Autodesk Fusion 360 part; units mm, degrees
note: some values were not read from the file. Set by a fixed rule: which face or edge a step refers to.
(part 2 of 4)
sketch "Sketch39" plane through (-432.6941, 0, 0) normal (-1, 0, 0) x (0, -1, 0)
  circle A0 centre (25, -180) radius 4
  circle A1 centre (50, 175) radius 4
  circle A2 centre (25, 170) radius 4
  circle A3 centre (50, -175) radius 4
  circle A4 centre (75, 180) radius 4
  circle A5 centre (75, -170) radius 4
  arc A6 (0, 125.6014) -> (0, 130.6014) centre (0, 128.1014) ccw
  line L0 (0, 125.6014) -> (-10, 125.6014)
  line L1 (-10, 125.6014) -> (-10, 18.1014)
  line L2 (-10, 18.1014) -> (0, 18.1014)
  arc A7 (0, 13.1014) -> (0, 18.1014) centre (0, 15.6014) ccw
  line L3 (0, 13.1014) -> (0, -6.8986)
  arc A8 (0, -11.8986) -> (0, -6.8986) centre (0, -9.3986) ccw
  line L4 (0, -11.8986) -> (-10, -11.8986)
  line L5 (-10, -11.8986) -> (-10, -119.3986)
  line L6 (-10, -119.3986) -> (0, -119.3986)
  arc A9 (0, -124.3986) -> (0, -119.3986) centre (0, -121.8986) ccw
  line L7 (0, -124.3986) -> (0, -144.3986)
  arc A10 (0, -149.3986) -> (0, -144.3986) centre (0, -146.8986) ccw
  line L8 (0, -149.3986) -> (-10, -149.3986)
  line L9 (-10, -149.3986) -> (-10, -256.3488)
  line L10 (-10, -256.3488) -> (30, -256.3488)
  line L11 (30, -256.3488) -> (30, -246.3488)
  arc A11 (35, -246.3488) -> (30, -246.3488) centre (32.5, -246.3488) ccw
  line L12 (35, -246.3488) -> (55, -246.3488)
  arc A12 (60, -246.3488) -> (55, -246.3488) centre (57.5, -246.3488) ccw
  line L13 (60, -246.3488) -> (60, -256.3488)
  line L14 (60, -256.3488) -> (100, -256.3488)
  line L15 (100, -256.3488) -> (100, 273.6512)
  line L16 (100, 273.6512) -> (60, 273.6512)
  line L17 (60, 273.6512) -> (60, 263.6512)
  arc A13 (55, 263.6512) -> (60, 263.6512) centre (57.5, 263.6512) ccw
  line L18 (55, 263.6512) -> (35, 263.6512)
  arc A14 (30, 263.6512) -> (35, 263.6512) centre (32.5, 263.6512) ccw
  line L19 (30, 263.6512) -> (30, 273.6512)
  line L20 (30, 273.6512) -> (-10, 273.6512)
  line L21 (-10, 273.6512) -> (-10, 155.6014)
  line L22 (-10, 155.6014) -> (0, 155.6014)
  arc A15 (0, 150.6014) -> (0, 155.6014) centre (0, 153.1014) ccw
  line L23 (0, 150.6014) -> (0, 140.6014)
  arc A16 (0, 135.6014) -> (0, 140.6014) centre (0, 138.1014) ccw
  line L24 (0, 135.6014) -> (0, 130.6014)
  line L25 (0, 140.6014) -> (2.5, 140.6014)
  line L26 (2.5, 140.6014) -> (2.5, 134.5426)
  line L27 (2.5, 134.5426) -> (0, 134.5426)
  line L28 (0, 134.5426) -> (0, 140.6014)
  constraint horizontal L25
  constraint vertical L26
  constraint horizontal L27
  constraint vertical L28
  constraint coincident L23.end A16.end
extrude "Extrude20" add sketch "Sketch39" against normal blind 10 contours A16 L28 bodies 3
sketch "Sketch40" plane through (-142.6941, 0, 0) normal (-1, 0, 0) x (0, -1, 0)
  line L0 (0, 135.6014) -> (0, 130.6014)
  arc A0 (0, 125.6014) -> (0, 130.6014) centre (0, 128.1014) ccw
  line L1 (0, 125.6014) -> (-10, 125.6014)
  line L2 (-10, 125.6014) -> (-10, 18.1014)
  line L3 (-10, 18.1014) -> (0, 18.1014)
  arc A1 (0, 13.1014) -> (0, 18.1014) centre (0, 15.6014) ccw
  line L4 (0, 13.1014) -> (0, -6.8986)
  arc A2 (0, -11.8986) -> (0, -6.8986) centre (0, -9.3986) ccw
  line L5 (0, -11.8986) -> (-10, -11.8986)
  line L6 (-10, -11.8986) -> (-10, -119.3986)
  line L7 (-10, -119.3986) -> (0, -119.3986)
  arc A3 (0, -124.3986) -> (0, -119.3986) centre (0, -121.8986) ccw
  line L8 (0, -124.3986) -> (0, -144.3986)
  arc A4 (0, -149.3986) -> (0, -144.3986) centre (0, -146.8986) ccw
  line L9 (0, -149.3986) -> (-10, -149.3986)
  line L10 (-10, -149.3986) -> (-10, -256.3488)
  line L11 (-10, -256.3488) -> (30, -256.3488)
  line L12 (30, -256.3488) -> (30, -246.3488)
  arc A5 (35, -246.3488) -> (30, -246.3488) centre (32.5, -246.3488) ccw
  line L13 (35, -246.3488) -> (55, -246.3488)
  arc A6 (60, -246.3488) -> (55, -246.3488) centre (57.5, -246.3488) ccw
  line L14 (60, -246.3488) -> (60, -256.3488)
  line L15 (60, -256.3488) -> (100, -256.3488)
  line L16 (100, -256.3488) -> (100, 273.6512)
  line L17 (100, 273.6512) -> (60, 273.6512)
  line L18 (60, 273.6512) -> (60, 263.6512)
  arc A7 (55, 263.6512) -> (60, 263.6512) centre (57.5, 263.6512) ccw
  line L19 (55, 263.6512) -> (35, 263.6512)
  arc A8 (30, 263.6512) -> (35, 263.6512) centre (32.5, 263.6512) ccw
  line L20 (30, 263.6512) -> (30, 273.6512)
  line L21 (30, 273.6512) -> (-10, 273.6512)
  line L22 (-10, 273.6512) -> (-10, 155.6014)
  line L23 (-10, 155.6014) -> (0, 155.6014)
  arc A9 (0, 150.6014) -> (0, 155.6014) centre (0, 153.1014) ccw
  line L24 (0, 150.6014) -> (0, 140.6014)
  arc A10 (0, 135.6014) -> (0, 140.6014) centre (0, 138.1014) ccw
  circle A11 centre (75, -170) radius 4
  circle A12 centre (75, 180) radius 4
  circle A13 centre (50, -175) radius 4
  circle A14 centre (25, 170) radius 4
  circle A15 centre (50, 175) radius 4
  circle A16 centre (25, -180) radius 4
  line L25 (0, 140.6014) -> (7, 140.6014)
  line L26 (7, 140.6014) -> (7, 132.6014)
  line L27 (7, 132.6014) -> (0, 132.6014)
  line L28 (0, 132.6014) -> (0, 140.6014)
  constraint horizontal L25
  constraint vertical L26
  constraint horizontal L27
  constraint vertical L28
  constraint coincident L24.end A10.end
extrude "Extrude21" add sketch "Sketch40" against normal blind 10 contours A10 L28 bodies 2
sketch "Sketch41" plane through (0, 0, 0) normal (0, -1, 0) x (1, 0, 0)
  line L0 (-332.6941, 163.1014) -> (-342.6941, 163.1014)
  line L1 (-342.6941, 163.1014) -> (-342.6941, 213.1014)
  line L2 (-342.6941, 213.1014) -> (-332.6941, 213.1014)
  line L3 (-332.6941, 213.1014) -> (-332.6941, 163.1014)
  point P0 (-332.6941, 163.1014)
  dimension "d245" = 10
  dimension "d246" = 50
  constraint horizontal L0
  constraint vertical L1
  constraint horizontal L2
  constraint vertical L3
  constraint coincident P0 L0.start
  measures "d245" distance of P0 L0.end
  measures "d246" distance of P0 L2.end
extrude "Extrude22" add sketch "Sketch41" along normal blind 70 separate body makes body 5
sketch "Sketch42" plane through (-332.6941, 0, 0) normal (1, 0, 0) x (0, 1, 0)
  line L0 (0, 163.1014) -> (0, 213.1014)
  line L1 (0, 213.1014) -> (-70, 213.1014)
  line L2 (-70, 213.1014) -> (-70, 163.1014)
  line L3 (-70, 163.1014) -> (0, 163.1014)
  line L4 (0, 198.1014) -> (10, 198.1014)
  line L5 (10, 198.1014) -> (10, 178.1014)
  line L6 (10, 178.1014) -> (0, 178.1014)
  line L7 (0, 178.1014) -> (0, 198.1014)
  line L8 (0, 193.1014) -> (0, 183.1014)
  line L9 (-70, 223.1014) -> (-65, 223.1014)
  line L10 (-65, 223.1014) -> (-65, 213.1014)
  line L11 (-65, 213.1014) -> (-70, 213.1014)
  line L12 (-70, 213.1014) -> (-70, 223.1014)
  dimension "d249" = 10
  dimension "d250" = 20
  dimension "d251" = 5
  dimension "d252" = 10
  constraint horizontal L4
  constraint vertical L5
  constraint horizontal L6
  constraint vertical L7
  constraint midpoint L7 L8
  constraint horizontal L9
  constraint vertical L10
  constraint horizontal L11
  constraint vertical L12
  constraint coincident L1.end L2.start
  measures "d249" distance of L4.start L4.end
  measures "d250" distance of L4.start L6.end
  measures "d251" distance of L9.start L9.end
  measures "d252" distance of L9.start L1.end
extrude "Extrude23" add sketch "Sketch42" against normal blind 10 contours L0 L4 L5 L6 L7 L8 | L1 L9 L10 L11 L12 bodies 5
sketch "Sketch43" plane through (-332.6941, 0, 0) normal (1, 0, 0) x (0, 1, 0)
  line L0 (0, 198.1014) -> (0, 213.1014)
  line L1 (0, 213.1014) -> (-65, 213.1014)
  line L2 (-65, 213.1014) -> (-65, 223.1014)
  line L3 (-65, 223.1014) -> (-70, 223.1014)
  line L4 (-70, 223.1014) -> (-70, 163.1014)
  line L5 (-70, 163.1014) -> (0, 163.1014)
  line L6 (0, 163.1014) -> (0, 178.1014)
  line L7 (0, 178.1014) -> (10, 178.1014)
  line L8 (10, 178.1014) -> (10, 198.1014)
  line L9 (10, 198.1014) -> (0, 198.1014)
  circle A0 centre (0, 200.6014) radius 2.5
  circle A1 centre (0, 175.6014) radius 2.5
  circle A2 centre (-62.5, 213.1014) radius 2.5
  line L10 (-5.4259, 163.1014) -> (-70, 190)
  line L11 (-70, 163.1014) -> (-70, 190)
  line L12 (-70, 163.1014) -> (-5.4259, 163.1014)
  dimension "d255" = 5
  dimension "d256" = 5
  dimension "d257" = 5
  constraint coincident L0.start A0
  constraint coincident L6.end A1
  constraint coincident L1.end A2
  constraint coincident L5 L10.start
  constraint coincident L4 L10.end
  constraint coincident L4.end L5.start
  measures "d255" diameter of A0
  measures "d256" diameter of A1
  measures "d257" diameter of A2
extrude "Extrude24" cut sketch "Sketch43" against normal blind 10 contours L0 A0 | L1 A2 | L6 A1 | L4 L5 L10 L11 L12 picked at (-0.8152, 201.2122) picked at (-62.5623, 212.2704) picked at (-0.8999, 175.0818) bodies 5
copy_body "CopyPasteBodies2" bodies 5 makes body 6
move_body "Move3" bodies 6 to x (1, 0, 0) y (0, 1, 0) z (0, 0, 1) at (100, 0, 0)
move_body "Move4" bodies 6 to x (1, 0, 0) y (0, 1, 0) z (0, 0, 1) at (10, 0, 0)
sketch "Sketch44" plane through (0, 0, 0) normal (0, -1, 0) x (1, 0, 0)
sketch "Sketch45" plane through (0, 0, 263.1014) normal (0, 0, 1) x (-1, 0, 0)
  line L0 (357.6941, 0) -> (332.6941, 0)
  line L1 (332.6941, 0) -> (332.6941, -10)
  line L2 (332.6941, -10) -> (357.6941, -10)
  line L3 (357.6941, -10) -> (357.6941, 0)
  line L4 (432.6941, -10) -> (132.6941, -10)
  line L5 (132.6941, -10) -> (132.6941, 100)
  line L6 (132.6941, 100) -> (432.6941, 100)
  line L7 (432.6941, 100) -> (432.6941, -10)
  line L8 (432.6941, 100) -> (422.6941, 100)
  line L9 (422.6941, 100) -> (422.6941, 55)
  line L10 (422.6941, 55) -> (432.6941, 55)
  line L11 (432.6941, 55) -> (432.6941, 100)
  line L12 (432.6941, -10) -> (442.6941, -10)
  line L13 (442.6941, -10) -> (442.6941, -55)
  line L14 (442.6941, -55) -> (432.6941, -55)
  line L15 (432.6941, -55) -> (432.6941, -10)
  line L16 (132.6941, -10) -> (142.6941, -10)
  line L17 (142.6941, -10) -> (142.6941, 35)
  line L18 (142.6941, 35) -> (132.6941, 35)
  line L19 (132.6941, 35) -> (132.6941, -10)
  line L20 (132.6941, 100) -> (142.6941, 100)
  line L21 (142.6941, 100) -> (142.6941, 55)
  line L22 (142.6941, 55) -> (132.6941, 55)
  line L23 (132.6941, 55) -> (132.6941, 100)
  line L24 (392.6941, 0) -> (362.6941, 0)
  line L25 (362.6941, 0) -> (362.6941, -10)
  line L26 (362.6941, -10) -> (392.6941, -10)
  line L27 (392.6941, -10) -> (392.6941, 0)
  line L28 (202.6941, 0) -> (172.6941, 0)
  line L29 (172.6941, 0) -> (172.6941, -10)
  line L30 (172.6941, -10) -> (202.6941, -10)
  line L31 (202.6941, -10) -> (202.6941, 0)
  point P0 (432.6941, -10)
  point P1 (392.6941, 0)
  point P2 (202.6941, 0)
  dimension "d260" = 10
  dimension "d261" = 45
  dimension "d262" = 10
  dimension "d263" = 45
  dimension "d264" = 10
  dimension "d265" = 45
  dimension "d266" = 10
  dimension "d267" = 45
  dimension "d268" = 30
  dimension "d269" = 10
  dimension "d270" = 30
  dimension "d271" = 10
  constraint horizontal L4
  constraint vertical L5
  constraint horizontal L6
  constraint vertical L7
  constraint coincident P0 L4.start
  constraint horizontal L8
  constraint vertical L9
  constraint horizontal L10
  constraint vertical L11
  constraint horizontal L12
  constraint vertical L13
  constraint horizontal L14
  constraint vertical L15
  constraint horizontal L16
  constraint vertical L17
  constraint horizontal L18
  constraint vertical L19
  constraint horizontal L20
  constraint vertical L21
  constraint horizontal L22
  constraint vertical L23
  constraint horizontal L24
  constraint vertical L25
  constraint horizontal L26
  constraint vertical L27
  constraint coincident P1 L24.start
  constraint horizontal L28
  constraint vertical L29
  constraint horizontal L30
  constraint vertical L31
  constraint coincident P2 L28.start
  measures "d260" distance of L6.end L8.end
  measures "d261" distance of L6.end L10.end
  measures "d262" distance of P0 L12.end
  measures "d263" distance of P0 L14.end
  measures "d264" distance of L4.end L16.end
  measures "d265" distance of L4.end L18.end
  measures "d266" distance of L5.end L20.end
  measures "d267" distance of L5.end L22.end
  measures "d268" distance of P1 L24.end
  measures "d269" distance of P1 L26.end
  measures "d270" distance of P2 L28.end
  measures "d271" distance of P2 L30.end
extrude "Extrude25" add sketch "Sketch45" along normal blind 10 separate body contours L0 L1 L3 L4 L5 L6 L7 L9 L10 L17 L18 L21 L22 L24 L25 L27 L28 L29 L31 makes body 7
sketch "Sketch46" plane through (0, 0, 273.1014) normal (0, 0, 1) x (-1, 0, 0)
  line L0 (142.6941, 100) -> (142.6941, 55)
  line L1 (142.6941, 55) -> (132.6941, 55)
  line L2 (132.6941, 55) -> (132.6941, 35)
  line L3 (132.6941, 35) -> (142.6941, 35)
  line L4 (142.6941, 35) -> (142.6941, -10)
  line L5 (142.6941, -10) -> (172.6941, -10)
  line L6 (172.6941, -10) -> (172.6941, 0)
  line L7 (172.6941, 0) -> (202.6941, 0)
  line L8 (202.6941, 0) -> (202.6941, -10)
  line L9 (202.6941, -10) -> (332.6941, -10)
  line L10 (332.6941, -10) -> (332.6941, 0)
  line L11 (332.6941, 0) -> (357.6941, 0)
  line L12 (357.6941, 0) -> (357.6941, -10)
  line L13 (357.6941, -10) -> (362.6941, -10)
  line L14 (362.6941, -10) -> (362.6941, 0)
  line L15 (362.6941, 0) -> (392.6941, 0)
  line L16 (392.6941, 0) -> (392.6941, -10)
  line L17 (392.6941, -10) -> (432.6941, -10)
  line L18 (432.6941, -10) -> (432.6941, 55)
  line L19 (432.6941, 55) -> (422.6941, 55)
  line L20 (422.6941, 55) -> (422.6941, 100)
  line L21 (422.6941, 100) -> (142.6941, 100)
  line L22 (357.6941, -10) -> (332.6941, -10)
  line L23 (332.6941, -10) -> (332.6941, 0)
  line L24 (332.6941, 0) -> (357.6941, 0)
  line L25 (357.6941, 0) -> (357.6941, -10)
  constraint horizontal L22
  constraint vertical L23
  constraint horizontal L24
  constraint vertical L25
  constraint coincident L10.end L11.start
  constraint coincident L12.end L13.start
extrude "Extrude26" add sketch "Sketch46" against normal blind 10 contours L10 L11 L12 L22 L23 L24 L25 bodies 7
sketch "Sketch47" plane through (0, 0, 273.1014) normal (0, 0, 1) x (-1, 0, 0)
  line L0 (142.6941, 100) -> (142.6941, 55)
  line L1 (142.6941, 55) -> (132.6941, 55)
  line L2 (132.6941, 55) -> (132.6941, 35)
  line L3 (132.6941, 35) -> (142.6941, 35)
  line L4 (142.6941, 35) -> (142.6941, -10)
  line L5 (142.6941, -10) -> (172.6941, -10)
  line L6 (172.6941, -10) -> (172.6941, 0)
  line L7 (172.6941, 0) -> (202.6941, 0)
  line L8 (202.6941, 0) -> (202.6941, -10)
  line L9 (202.6941, -10) -> (362.6941, -10)
  line L10 (362.6941, -10) -> (362.6941, 0)
  line L11 (362.6941, 0) -> (392.6941, 0)
  line L12 (392.6941, 0) -> (392.6941, -10)
  line L13 (392.6941, -10) -> (432.6941, -10)
  line L14 (432.6941, -10) -> (432.6941, 55)
  line L15 (432.6941, 55) -> (422.6941, 55)
  line L16 (422.6941, 55) -> (422.6941, 100)
  line L17 (422.6941, 100) -> (142.6941, 100)
  line L18 (142.6941, 30) -> (132.6941, 30)
  line L19 (132.6941, 30) -> (132.6941, 60)
  line L20 (132.6941, 60) -> (142.6941, 60)
  line L21 (142.6941, 60) -> (142.6941, 30)
  dimension "d276" = 10
  dimension "d277" = 30
  constraint horizontal L18
  constraint vertical L19
  constraint horizontal L20
  constraint vertical L21
  constraint midpoint L2 L19
  measures "d276" distance of L18.start L18.end
  measures "d277" distance of L18.start L20.end
extrude "Extrude27" add sketch "Sketch47" against normal blind 10 contours L0 L1 L19 L20 L21 | L3 L4 L18 L19 L21 bodies 7
sketch "Sketch48" plane through (0, 0, 273.1014) normal (0, 0, 1) x (-1, 0, 0)
  line L0 (142.6941, 100) -> (142.6941, 60)
  line L1 (142.6941, 60) -> (132.6941, 60)
  line L2 (132.6941, 60) -> (132.6941, 30)
  line L3 (132.6941, 30) -> (142.6941, 30)
  line L4 (142.6941, 30) -> (142.6941, -10)
  line L5 (142.6941, -10) -> (172.6941, -10)
  line L6 (172.6941, -10) -> (172.6941, 0)
  line L7 (172.6941, 0) -> (202.6941, 0)
  line L8 (202.6941, 0) -> (202.6941, -10)
  line L9 (202.6941, -10) -> (362.6941, -10)
  line L10 (362.6941, -10) -> (362.6941, 0)
  line L11 (362.6941, 0) -> (392.6941, 0)
  line L12 (392.6941, 0) -> (392.6941, -10)
  line L13 (392.6941, -10) -> (432.6941, -10)
  line L14 (432.6941, -10) -> (432.6941, 55)
  line L15 (432.6941, 55) -> (422.6941, 55)
  line L16 (422.6941, 55) -> (422.6941, 100)
  line L17 (422.6941, 100) -> (142.6941, 100)
  line L18 (432.6941, -10) -> (422.6941, -10)
  line L19 (422.6941, -10) -> (422.6941, 30)
  line L20 (422.6941, 30) -> (432.6941, 30)
  line L21 (432.6941, 30) -> (432.6941, -10)
  dimension "d280" = 10
  dimension "d281" = 40
  constraint horizontal L18
  constraint vertical L19
  constraint horizontal L20
  constraint vertical L21
  constraint coincident L13.end L14.start
  measures "d280" distance of L13.end L18.end
  measures "d281" distance of L13.end L20.end
extrude "Extrude28" cut sketch "Sketch48" against normal blind 10 contours L13 L14 L18 L19 L20 L21 bodies 7
sketch "Sketch49" plane through (0, 0, 273.1014) normal (0, 0, 1) x (-1, 0, 0)
  line L0 (422.6941, -10) -> (422.6941, 30)
  line L1 (422.6941, 30) -> (432.6941, 30)
  line L2 (432.6941, 30) -> (432.6941, 55)
  line L3 (432.6941, 55) -> (422.6941, 55)
  line L4 (422.6941, 55) -> (422.6941, 100)
  line L5 (422.6941, 100) -> (142.6941, 100)
  line L6 (142.6941, 100) -> (142.6941, 60)
  line L7 (142.6941, 60) -> (132.6941, 60)
  line L8 (132.6941, 60) -> (132.6941, 30)
  line L9 (132.6941, 30) -> (142.6941, 30)
  line L10 (142.6941, 30) -> (142.6941, -10)
  line L11 (142.6941, -10) -> (172.6941, -10)
  line L12 (172.6941, -10) -> (172.6941, 0)
  line L13 (172.6941, 0) -> (202.6941, 0)
  line L14 (202.6941, 0) -> (202.6941, -10)
  line L15 (202.6941, -10) -> (362.6941, -10)
  line L16 (362.6941, -10) -> (362.6941, 0)
  line L17 (362.6941, 0) -> (392.6941, 0)
  line L18 (392.6941, 0) -> (392.6941, -10)
  line L19 (392.6941, -10) -> (422.6941, -10)
  line L20 (422.6941, 55) -> (432.6941, 55)
  line L21 (432.6941, 55) -> (432.6941, 60)
  line L22 (432.6941, 60) -> (422.6941, 60)
  line L23 (422.6941, 60) -> (422.6941, 55)
  dimension "d284" = 10
  dimension "d285" = 5
  constraint horizontal L20
  constraint vertical L21
  constraint horizontal L22
  constraint vertical L23
  constraint coincident L3.end L4.start
  measures "d284" distance of L3.end L2.end
  measures "d285" distance of L3.end L22.end
extrude "Extrude29" add sketch "Sketch49" against normal blind 10 contours L3 L4 L20 L21 L22 L23 bodies 7
sketch "Sketch50" plane through (0, 0, 273.1014) normal (0, 0, 1) x (-1, 0, 0)
  line L0 (422.6941, -10) -> (422.6941, 30)
  line L1 (422.6941, 30) -> (432.6941, 30)
  line L2 (432.6941, 30) -> (432.6941, 60)
  line L3 (432.6941, 60) -> (422.6941, 60)
  line L4 (422.6941, 60) -> (422.6941, 100)
  line L5 (422.6941, 100) -> (142.6941, 100)
  line L6 (142.6941, 100) -> (142.6941, 60)
  line L7 (142.6941, 60) -> (132.6941, 60)
  line L8 (132.6941, 60) -> (132.6941, 30)
  line L9 (132.6941, 30) -> (142.6941, 30)
  line L10 (142.6941, 30) -> (142.6941, -10)
  line L11 (142.6941, -10) -> (172.6941, -10)
  line L12 (172.6941, -10) -> (172.6941, 0)
  line L13 (172.6941, 0) -> (202.6941, 0)
  line L14 (202.6941, 0) -> (202.6941, -10)
  line L15 (202.6941, -10) -> (362.6941, -10)
  line L16 (362.6941, -10) -> (362.6941, 0)
  line L17 (362.6941, 0) -> (392.6941, 0)
  line L18 (392.6941, 0) -> (392.6941, -10)
  line L19 (392.6941, -10) -> (422.6941, -10)
  circle A0 centre (365.1941, 0.0132) radius 2.5
  circle A1 centre (390.1941, 0) radius 2.5
  circle A2 centre (422.6941, 27.5) radius 2.5
  circle A3 centre (422.6941, 62.5) radius 2.5
  dimension "d288" = 5
  dimension "d289" = 5
  dimension "d290" = 5
  dimension "d291" = 5
  constraint coincident L16.end A0
  constraint coincident L17.end A1
  constraint coincident L0.end A2
  constraint coincident L3.end A3
  measures "d288" diameter of A0
  measures "d289" diameter of A1
  measures "d290" diameter of A2
  measures "d291" diameter of A3
extrude "Extrude30" cut sketch "Sketch50" against normal blind 10 contours L0 A2 | L17 A1 | L17 A0 | L4 A3 picked at (421.9184, 27.8045) picked at (390.805, 0.8152) picked at (365.5655, 1.494) picked at (421.9184, 62.1955) bodies 7
sketch "Sketch51" plane through (0, 0, 273.1014) normal (0, 0, 1) x (-1, 0, 0)
  arc A0 (367.694, 0) -> (362.6941, 0) centre (365.1941, 0.0132) ccw
  line L0 (367.694, 0) -> (387.6941, 0)
  arc A1 (392.6941, 0) -> (387.6941, 0) centre (390.1941, 0) ccw
  line L1 (392.6941, 0) -> (392.6941, -10)
  line L2 (392.6941, -10) -> (422.6941, -10)
  line L3 (422.6941, -10) -> (422.6941, 25)
  arc A2 (422.6941, 30) -> (422.6941, 25) centre (422.6941, 27.5) ccw
  line L4 (422.6941, 30) -> (432.6941, 30)
  line L5 (432.6941, 30) -> (432.6941, 60)
  line L6 (432.6941, 60) -> (422.6941, 60)
  arc A3 (422.6941, 65) -> (422.6941, 60) centre (422.6941, 62.5) ccw
  line L7 (422.6941, 65) -> (422.6941, 100)
  line L8 (422.6941, 100) -> (142.6941, 100)
  line L9 (142.6941, 100) -> (142.6941, 60)
  line L10 (142.6941, 60) -> (132.6941, 60)
  line L11 (132.6941, 60) -> (132.6941, 30)
  line L12 (132.6941, 30) -> (142.6941, 30)
  line L13 (142.6941, 30) -> (142.6941, -10)
  line L14 (142.6941, -10) -> (172.6941, -10)
  line L15 (172.6941, -10) -> (172.6941, 0)
  line L16 (172.6941, 0) -> (202.6941, 0)
  line L17 (202.6941, 0) -> (202.6941, -10)
  line L18 (202.6941, -10) -> (362.6941, -10)
  line L19 (362.6941, -10) -> (362.6941, 0)
  circle A4 centre (200.1941, 0) radius 2.5
  circle A5 centre (175.1941, 0) radius 2.5
  circle A6 centre (142.6941, 27.5) radius 2.5
  circle A7 centre (142.6941, 62.5) radius 2.5
  dimension "d294" = 5
  dimension "d295" = 5
  dimension "d296" = 5
  dimension "d297" = 5
  constraint coincident L16.end A4
  constraint coincident L15.end A5
  constraint coincident L12.end A6
  constraint coincident L9.end A7
  measures "d294" diameter of A4
  measures "d295" diameter of A5
  measures "d296" diameter of A6
  measures "d297" diameter of A7
extrude "Extrude31" cut sketch "Sketch51" against normal blind 10 contours L16 A4 | L16 A5 | L13 A6 | L9 A7 picked at (200.805, 0.8152) picked at (175.805, 0.8152) picked at (143.5189, 27.6186) picked at (143.7934, 63.0457) bodies 7
copy_body "CopyPasteBodies3" bodies 7 makes body 8
move_body "Move5" bodies 8 to x (1, 0, 0) y (0, 1, 0) z (0, 0, 1) at (0, 0, -520)
sketch "Sketch52" plane through (0, 10, 0) normal (0, 1, 0) x (-1, 0, 0)
  line L0 (142.6941, 120.6018) -> (142.6941, 23.1014)
  arc A0 (142.6941, 18.1014) -> (142.6941, 23.1014) centre (142.6941, 20.6014) ccw
  line L1 (142.6941, 18.1014) -> (132.6941, 18.1014)
  line L2 (132.6941, 18.1014) -> (132.6941, -11.8986)
  line L3 (132.6941, -11.8986) -> (142.6941, -11.8986)
  arc A1 (142.6941, -16.8986) -> (142.6941, -11.8986) centre (142.6941, -14.3986) ccw
  line L4 (142.6941, -16.8986) -> (142.6941, -114.3986)
  arc A2 (142.6941, -119.3986) -> (142.6941, -114.3986) centre (142.6941, -116.8986) ccw
  line L5 (142.6941, -119.3986) -> (132.6941, -119.3986)
  line L6 (132.6941, -119.3986) -> (132.6941, -149.3986)
  line L7 (132.6941, -149.3986) -> (142.6941, -149.3986)
  arc A3 (142.6941, -154.3986) -> (142.6941, -149.3986) centre (142.6941, -151.8986) ccw
  line L8 (142.6941, -154.3986) -> (142.6941, -256.8986)
  line L9 (142.6941, -256.8986) -> (422.6941, -256.8986)
  line L10 (422.6941, -256.8986) -> (422.6941, -154.3986)
  arc A4 (422.6941, -149.3986) -> (422.6941, -154.3986) centre (422.6941, -151.8986) ccw
  line L11 (422.6941, -149.3986) -> (432.6941, -149.3986)
  line L12 (432.6941, -149.3986) -> (432.6941, -119.3986)
  line L13 (432.6941, -119.3986) -> (422.6941, -119.3986)
  arc A5 (422.6941, -114.3986) -> (422.6941, -119.3986) centre (422.6941, -116.8986) ccw
  line L14 (422.6941, -114.3986) -> (422.6941, -16.8986)
  arc A6 (422.6941, -11.8986) -> (422.6941, -16.8986) centre (422.6941, -14.3986) ccw
  line L15 (422.6941, -11.8986) -> (432.6941, -11.8986)
  line L16 (432.6941, -11.8986) -> (432.6941, 18.1014)
  line L17 (432.6941, 18.1014) -> (422.6941, 18.1014)
  arc A7 (422.6941, 23.1014) -> (422.6941, 18.1014) centre (422.6941, 20.6014) ccw
  line L18 (422.6941, 23.1014) -> (422.6941, 120.6038)
  arc A8 (422.8505, 125.6014) -> (422.6941, 120.6038) centre (422.7723, 123.1026) ccw
  line L19 (422.8505, 125.6014) -> (432.6941, 125.6014)
  line L20 (432.6941, 125.6014) -> (432.6941, 155.6014)
  line L21 (432.6941, 155.6014) -> (422.6941, 155.6014)
  arc A9 (422.6941, 160.6014) -> (422.6941, 155.6014) centre (422.6941, 158.1014) ccw
  line L22 (422.6941, 160.6014) -> (422.6941, 263.1014)
  line L23 (422.6941, 263.1014) -> (397.6941, 263.1014)
  arc A10 (392.6941, 263.1014) -> (397.6941, 263.1014) centre (395.1941, 263.1014) ccw
  line L24 (392.6941, 263.1014) -> (392.6941, 273.1014)
  line L25 (392.6941, 273.1014) -> (362.6941, 273.1014)
  line L26 (362.6941, 273.1014) -> (362.6941, 263.1014)
  arc A11 (357.6941, 263.1014) -> (362.6941, 263.1014) centre (360.1941, 263.1014) ccw
  line L27 (357.6941, 263.1014) -> (332.6941, 263.1014)
  line L28 (332.6941, 263.1014) -> (332.6941, 198.1014)
  line L29 (332.6941, 198.1014) -> (342.6941, 198.1014)
  arc A12 (342.6941, 193.1014) -> (342.6941, 198.1014) centre (342.6941, 195.6014) ccw
  line L30 (342.6941, 193.1014) -> (342.6941, 183.1014)
  arc A13 (342.6941, 178.1014) -> (342.6941, 183.1014) centre (342.6941, 180.6014) ccw
  line L31 (342.6941, 178.1014) -> (332.6941, 178.1014)
  line L32 (332.6941, 178.1014) -> (332.6941, 163.1014)
  line L33 (332.6941, 163.1014) -> (232.6941, 163.1014)
  line L34 (232.6941, 163.1014) -> (232.6941, 178.1014)
  line L35 (232.6941, 178.1014) -> (222.6941, 178.1014)
  arc A14 (222.6941, 183.1014) -> (222.6941, 178.1014) centre (222.6941, 180.6014) ccw
  line L36 (222.6941, 183.1014) -> (222.6941, 193.1014)
  arc A15 (222.6941, 198.1014) -> (222.6941, 193.1014) centre (222.6941, 195.6014) ccw
  line L37 (222.6941, 198.1014) -> (232.6941, 198.1014)
  line L38 (232.6941, 198.1014) -> (232.6941, 263.1014)
  line L39 (232.6941, 263.1014) -> (207.6941, 263.1014)
  arc A16 (202.6941, 263.1014) -> (207.6941, 263.1014) centre (205.1941, 263.1014) ccw
  line L40 (202.6941, 263.1014) -> (202.6941, 273.1014)
  line L41 (202.6941, 273.1014) -> (172.6941, 273.1014)
  line L42 (172.6941, 273.1014) -> (172.6941, 263.1014)
  arc A17 (167.6941, 263.1014) -> (172.6941, 263.1014) centre (170.1941, 263.1014) ccw
  line L43 (167.6941, 263.1014) -> (142.6941, 263.1014)
  line L44 (142.6941, 263.1014) -> (142.6941, 160.6009)
  arc A18 (142.6941, 155.6018) -> (142.6941, 160.6009) centre (142.6471, 158.1014) ccw
  line L45 (142.6941, 155.6018) -> (142.6941, 155.5705)
  line L46 (142.6941, 155.5705) -> (132.6941, 155.5705)
  line L47 (132.6941, 155.5705) -> (132.6941, 125.6014)
  line L48 (132.6941, 125.6014) -> (142.6941, 125.6014)
  line L49 (142.6941, 125.6014) -> (142.6941, 125.6009)
  arc A19 (142.6941, 120.6018) -> (142.6941, 125.6009) centre (142.6471, 123.1014) ccw
  line L50 (365.1941, 98.1014) -> (365.1941, -66.8986)
  line L51 (365.1941, -66.8986) -> (200.1941, -66.8986)
  line L52 (200.1941, -66.8986) -> (200.1941, 98.1014)
  line L53 (200.1941, 98.1014) -> (365.1941, 98.1014)
  line L54 (142.6941, -247.1839) -> (177.6941, -247.1839)
  line L55 (177.6941, -247.1839) -> (177.6941, -257.1839)
  line L56 (177.6941, -257.1839) -> (142.6941, -257.1839)
  line L57 (142.6941, -257.1839) -> (142.6941, -247.1839)
  line L58 (197.8622, -246.9544) -> (367.8622, -246.9544)
  line L59 (367.8622, -246.9544) -> (367.8622, -256.9544)
  line L60 (367.8622, -256.9544) -> (197.8622, -256.9544)
  line L61 (197.8622, -256.9544) -> (197.8622, -246.9544)
  line L62 (422.6941, -256.8986) -> (387.6941, -256.8986)
  line L63 (387.6941, -256.8986) -> (387.6941, -246.8986)
  line L64 (387.6941, -246.8986) -> (422.6941, -246.8986)
  line L65 (422.6941, -246.8986) -> (422.6941, -256.8986)
  dimension "d300" = 35
  dimension "d301" = 10
  dimension "d302" = 170
  dimension "d303" = 10
  dimension "d304" = 35
  dimension "d305" = 10
  constraint horizontal L54
  constraint vertical L55
  constraint horizontal L56
  constraint vertical L57
  constraint coincident L8 L54.start
  constraint horizontal L58
  constraint vertical L59
  constraint horizontal L60
  constraint vertical L61
  constraint horizontal L62
  constraint vertical L63
  constraint horizontal L64
  constraint vertical L65
  constraint coincident L9.end L10.start
  measures "d300" distance of L54.start L54.end
  measures "d301" distance of L54.start L56.end
  measures "d302" distance of L58.start L58.end
  measures "d303" distance of L58.start L60.end
  measures "d304" distance of L9.end L62.end
  measures "d305" distance of L9.end L64.end
extrude "Extrude32" cut sketch "Sketch52" against normal blind 10 contours L8 L9 L54 L55 L57 | L9 L58 L59 L61 | L9 L10 L62 L63 L64 L65 bodies 1
sketch "Sketch53" plane through (0, 0, 0) normal (0, -1, 0) x (1, 0, 0)
  line L0 (-365.1941, -66.8986) -> (-365.1941, 98.1014)
  line L1 (-365.1941, 98.1014) -> (-200.1941, 98.1014)
  line L2 (-200.1941, 98.1014) -> (-200.1941, -66.8986)
  line L3 (-200.1941, -66.8986) -> (-365.1941, -66.8986)
  line L4 (-422.6941, -246.8986) -> (-387.6941, -246.8986)
  line L5 (-387.6941, -246.8986) -> (-387.6941, -256.8986)
  line L6 (-387.6941, -256.8986) -> (-367.8622, -256.8986)
  line L7 (-367.8622, -256.8986) -> (-367.8622, -246.9544)
  line L8 (-367.8622, -246.9544) -> (-197.8622, -246.9544)
  line L9 (-197.8622, -246.9544) -> (-197.8622, -256.8986)
  line L10 (-197.8622, -256.8986) -> (-177.6941, -256.8986)
  line L11 (-177.6941, -256.8986) -> (-177.6941, -247.1839)
  line L12 (-177.6941, -247.1839) -> (-142.6941, -247.1839)
  line L13 (-142.6941, -247.1839) -> (-142.6941, -154.3986)
  arc A0 (-142.6941, -149.3986) -> (-142.6941, -154.3986) centre (-142.6941, -151.8986) ccw
  line L14 (-142.6941, -149.3986) -> (-132.6941, -149.3986)
  line L15 (-132.6941, -149.3986) -> (-132.6941, -119.3986)
  line L16 (-132.6941, -119.3986) -> (-142.6941, -119.3986)
  arc A1 (-142.6941, -114.3986) -> (-142.6941, -119.3986) centre (-142.6941, -116.8986) ccw
  line L17 (-142.6941, -114.3986) -> (-142.6941, -16.8986)
  arc A2 (-142.6941, -11.8986) -> (-142.6941, -16.8986) centre (-142.6941, -14.3986) ccw
  line L18 (-142.6941, -11.8986) -> (-132.6941, -11.8986)
  line L19 (-132.6941, -11.8986) -> (-132.6941, 18.1014)
  line L20 (-132.6941, 18.1014) -> (-142.6941, 18.1014)
  arc A3 (-142.6941, 23.1014) -> (-142.6941, 18.1014) centre (-142.6941, 20.6014) ccw
  line L21 (-142.6941, 23.1014) -> (-142.6941, 120.6018)
  arc A4 (-142.6941, 125.6009) -> (-142.6941, 120.6018) centre (-142.6471, 123.1014) ccw
  line L22 (-142.6941, 125.6009) -> (-142.6941, 125.6014)
  line L23 (-142.6941, 125.6014) -> (-132.6941, 125.6014)
  line L24 (-132.6941, 125.6014) -> (-132.6941, 155.5705)
  line L25 (-132.6941, 155.5705) -> (-142.6941, 155.5705)
  line L26 (-142.6941, 155.5705) -> (-142.6941, 155.6018)
  arc A5 (-142.6941, 160.6009) -> (-142.6941, 155.6018) centre (-142.6471, 158.1014) ccw
  line L27 (-142.6941, 160.6009) -> (-142.6941, 263.1014)
  line L28 (-142.6941, 263.1014) -> (-167.6941, 263.1014)
  arc A6 (-172.6941, 263.1014) -> (-167.6941, 263.1014) centre (-170.1941, 263.1014) ccw
  line L29 (-172.6941, 263.1014) -> (-172.6941, 273.1014)
  line L30 (-172.6941, 273.1014) -> (-202.6941, 273.1014)
  line L31 (-202.6941, 273.1014) -> (-202.6941, 263.1014)
  arc A7 (-207.6941, 263.1014) -> (-202.6941, 263.1014) centre (-205.1941, 263.1014) ccw
  line L32 (-207.6941, 263.1014) -> (-232.6941, 263.1014)
  line L33 (-232.6941, 263.1014) -> (-232.6941, 198.1014)
  line L34 (-232.6941, 198.1014) -> (-222.6941, 198.1014)
  arc A8 (-222.6941, 193.1014) -> (-222.6941, 198.1014) centre (-222.6941, 195.6014) ccw
  line L35 (-222.6941, 193.1014) -> (-222.6941, 183.1014)
  arc A9 (-222.6941, 178.1014) -> (-222.6941, 183.1014) centre (-222.6941, 180.6014) ccw
  line L36 (-222.6941, 178.1014) -> (-232.6941, 178.1014)
  line L37 (-232.6941, 178.1014) -> (-232.6941, 163.1014)
  line L38 (-232.6941, 163.1014) -> (-332.6941, 163.1014)
  line L39 (-332.6941, 163.1014) -> (-332.6941, 178.1014)
  line L40 (-332.6941, 178.1014) -> (-342.6941, 178.1014)
  arc A10 (-342.6941, 183.1014) -> (-342.6941, 178.1014) centre (-342.6941, 180.6014) ccw
  line L41 (-342.6941, 183.1014) -> (-342.6941, 193.1014)
  arc A11 (-342.6941, 198.1014) -> (-342.6941, 193.1014) centre (-342.6941, 195.6014) ccw
  line L42 (-342.6941, 198.1014) -> (-332.6941, 198.1014)
  line L43 (-332.6941, 198.1014) -> (-332.6941, 263.1014)
  line L44 (-332.6941, 263.1014) -> (-357.6941, 263.1014)
  arc A12 (-362.6941, 263.1014) -> (-357.6941, 263.1014) centre (-360.1941, 263.1014) ccw
  line L45 (-362.6941, 263.1014) -> (-362.6941, 273.1014)
  line L46 (-362.6941, 273.1014) -> (-392.6941, 273.1014)
  line L47 (-392.6941, 273.1014) -> (-392.6941, 263.1014)
  arc A13 (-397.6941, 263.1014) -> (-392.6941, 263.1014) centre (-395.1941, 263.1014) ccw
  line L48 (-397.6941, 263.1014) -> (-422.6941, 263.1014)
  line L49 (-422.6941, 263.1014) -> (-422.6941, 160.6014)
  arc A14 (-422.6941, 155.6014) -> (-422.6941, 160.6014) centre (-422.6941, 158.1014) ccw
  line L50 (-422.6941, 155.6014) -> (-432.6941, 155.6014)
  line L51 (-432.6941, 155.6014) -> (-432.6941, 125.6014)
  line L52 (-432.6941, 125.6014) -> (-422.8505, 125.6014)
  arc A15 (-422.6941, 120.6038) -> (-422.8505, 125.6014) centre (-422.7723, 123.1026) ccw
  line L53 (-422.6941, 120.6038) -> (-422.6941, 23.1014)
  arc A16 (-422.6941, 18.1014) -> (-422.6941, 23.1014) centre (-422.6941, 20.6014) ccw
  line L54 (-422.6941, 18.1014) -> (-432.6941, 18.1014)
  line L55 (-432.6941, 18.1014) -> (-432.6941, -11.8986)
  line L56 (-432.6941, -11.8986) -> (-422.6941, -11.8986)
  arc A17 (-422.6941, -16.8986) -> (-422.6941, -11.8986) centre (-422.6941, -14.3986) ccw
  line L57 (-422.6941, -16.8986) -> (-422.6941, -114.3986)
  arc A18 (-422.6941, -119.3986) -> (-422.6941, -114.3986) centre (-422.6941, -116.8986) ccw
  line L58 (-422.6941, -119.3986) -> (-432.6941, -119.3986)
  line L59 (-432.6941, -119.3986) -> (-432.6941, -149.3986)
  line L60 (-432.6941, -149.3986) -> (-422.6941, -149.3986)
  arc A19 (-422.6941, -154.3986) -> (-422.6941, -149.3986) centre (-422.6941, -151.8986) ccw
  line L61 (-422.6941, -154.3986) -> (-422.6941, -246.8986)
  circle A20 centre (-390.1941, -246.8986) radius 2.5
  circle A21 centre (-365.3622, -246.9544) radius 2.5
  circle A22 centre (-197.8622, -246.9544) radius 2.5
  circle A23 centre (-175.1941, -247.1839) radius 2.5
  dimension "d308" = 5
  dimension "d309" = 5
  dimension "d310" = 5
  dimension "d311" = 5
  constraint coincident L4.end A20
  constraint coincident L7.end A21
  constraint coincident L8.end L9.start
  constraint coincident L11.end A23
  measures "d308" diameter of A20
  measures "d309" diameter of A21
  measures "d310" diameter of A22
  measures "d311" diameter of A23
extrude "Extrude33" cut sketch "Sketch53" against normal blind 10 contours L4 A20 | L8 A21 | L12 A23 picked at (-390.1318, -246.0676) picked at (-365.2999, -246.1234) picked at (-175.1318, -246.3529) bodies 1
sketch "Sketch54" plane through (0, 0, 0) normal (0, -1, 0) x (1, 0, 0)
  line L0 (-365.1941, -66.8986) -> (-365.1941, 98.1014)
  line L1 (-365.1941, 98.1014) -> (-200.1941, 98.1014)
  line L2 (-200.1941, 98.1014) -> (-200.1941, -66.8986)
  line L3 (-200.1941, -66.8986) -> (-365.1941, -66.8986)
  arc A0 (-387.6941, -246.8986) -> (-392.6941, -246.8986) centre (-390.1941, -246.8986) ccw
  line L4 (-387.6941, -246.8986) -> (-387.6941, -256.8986)
  line L5 (-387.6941, -256.8986) -> (-367.8622, -256.8986)
  line L6 (-367.8622, -256.8986) -> (-367.8622, -246.9544)
  arc A1 (-362.8622, -246.9544) -> (-367.8622, -246.9544) centre (-365.3622, -246.9544) ccw
  line L7 (-362.8622, -246.9544) -> (-197.8622, -246.9544)
  line L8 (-197.8622, -246.9544) -> (-197.8622, -256.8986)
  line L9 (-197.8622, -256.8986) -> (-177.6941, -256.8986)
  line L10 (-177.6941, -256.8986) -> (-177.6941, -247.1839)
  arc A2 (-172.6941, -247.1839) -> (-177.6941, -247.1839) centre (-175.1941, -247.1839) ccw
  line L11 (-172.6941, -247.1839) -> (-142.6941, -247.1839)
  line L12 (-142.6941, -247.1839) -> (-142.6941, -154.3986)
  arc A3 (-142.6941, -149.3986) -> (-142.6941, -154.3986) centre (-142.6941, -151.8986) ccw
  line L13 (-142.6941, -149.3986) -> (-132.6941, -149.3986)
  line L14 (-132.6941, -149.3986) -> (-132.6941, -119.3986)
  line L15 (-132.6941, -119.3986) -> (-142.6941, -119.3986)
  arc A4 (-142.6941, -114.3986) -> (-142.6941, -119.3986) centre (-142.6941, -116.8986) ccw
  line L16 (-142.6941, -114.3986) -> (-142.6941, -16.8986)
  arc A5 (-142.6941, -11.8986) -> (-142.6941, -16.8986) centre (-142.6941, -14.3986) ccw
  line L17 (-142.6941, -11.8986) -> (-132.6941, -11.8986)
  line L18 (-132.6941, -11.8986) -> (-132.6941, 18.1014)
  line L19 (-132.6941, 18.1014) -> (-142.6941, 18.1014)
  arc A6 (-142.6941, 23.1014) -> (-142.6941, 18.1014) centre (-142.6941, 20.6014) ccw
  line L20 (-142.6941, 23.1014) -> (-142.6941, 120.6018)
  arc A7 (-142.6941, 125.6009) -> (-142.6941, 120.6018) centre (-142.6471, 123.1014) ccw
  line L21 (-142.6941, 125.6009) -> (-142.6941, 125.6014)
  line L22 (-142.6941, 125.6014) -> (-132.6941, 125.6014)
  line L23 (-132.6941, 125.6014) -> (-132.6941, 155.5705)
  line L24 (-132.6941, 155.5705) -> (-142.6941, 155.5705)
  line L25 (-142.6941, 155.5705) -> (-142.6941, 155.6018)
  arc A8 (-142.6941, 160.6009) -> (-142.6941, 155.6018) centre (-142.6471, 158.1014) ccw
  line L26 (-142.6941, 160.6009) -> (-142.6941, 263.1014)
  line L27 (-142.6941, 263.1014) -> (-167.6941, 263.1014)
  arc A9 (-172.6941, 263.1014) -> (-167.6941, 263.1014) centre (-170.1941, 263.1014) ccw
  line L28 (-172.6941, 263.1014) -> (-172.6941, 273.1014)
  line L29 (-172.6941, 273.1014) -> (-202.6941, 273.1014)
  line L30 (-202.6941, 273.1014) -> (-202.6941, 263.1014)
  arc A10 (-207.6941, 263.1014) -> (-202.6941, 263.1014) centre (-205.1941, 263.1014) ccw
  line L31 (-207.6941, 263.1014) -> (-232.6941, 263.1014)
  line L32 (-232.6941, 263.1014) -> (-232.6941, 198.1014)
  line L33 (-232.6941, 198.1014) -> (-222.6941, 198.1014)
  arc A11 (-222.6941, 193.1014) -> (-222.6941, 198.1014) centre (-222.6941, 195.6014) ccw
  line L34 (-222.6941, 193.1014) -> (-222.6941, 183.1014)
  arc A12 (-222.6941, 178.1014) -> (-222.6941, 183.1014) centre (-222.6941, 180.6014) ccw
  line L35 (-222.6941, 178.1014) -> (-232.6941, 178.1014)
  line L36 (-232.6941, 178.1014) -> (-232.6941, 163.1014)
  line L37 (-232.6941, 163.1014) -> (-332.6941, 163.1014)
  line L38 (-332.6941, 163.1014) -> (-332.6941, 178.1014)
  line L39 (-332.6941, 178.1014) -> (-342.6941, 178.1014)
  arc A13 (-342.6941, 183.1014) -> (-342.6941, 178.1014) centre (-342.6941, 180.6014) ccw
  line L40 (-342.6941, 183.1014) -> (-342.6941, 193.1014)
  arc A14 (-342.6941, 198.1014) -> (-342.6941, 193.1014) centre (-342.6941, 195.6014) ccw
  line L41 (-342.6941, 198.1014) -> (-332.6941, 198.1014)
  line L42 (-332.6941, 198.1014) -> (-332.6941, 263.1014)
  line L43 (-332.6941, 263.1014) -> (-357.6941, 263.1014)
  arc A15 (-362.6941, 263.1014) -> (-357.6941, 263.1014) centre (-360.1941, 263.1014) ccw
  line L44 (-362.6941, 263.1014) -> (-362.6941, 273.1014)
  line L45 (-362.6941, 273.1014) -> (-392.6941, 273.1014)
  line L46 (-392.6941, 273.1014) -> (-392.6941, 263.1014)
  arc A16 (-397.6941, 263.1014) -> (-392.6941, 263.1014) centre (-395.1941, 263.1014) ccw
  line L47 (-397.6941, 263.1014) -> (-422.6941, 263.1014)
  line L48 (-422.6941, 263.1014) -> (-422.6941, 160.6014)
  arc A17 (-422.6941, 155.6014) -> (-422.6941, 160.6014) centre (-422.6941, 158.1014) ccw
  line L49 (-422.6941, 155.6014) -> (-432.6941, 155.6014)
  line L50 (-432.6941, 155.6014) -> (-432.6941, 125.6014)
  line L51 (-432.6941, 125.6014) -> (-422.8505, 125.6014)
  arc A18 (-422.6941, 120.6038) -> (-422.8505, 125.6014) centre (-422.7723, 123.1026) ccw
  line L52 (-422.6941, 120.6038) -> (-422.6941, 23.1014)
  arc A19 (-422.6941, 18.1014) -> (-422.6941, 23.1014) centre (-422.6941, 20.6014) ccw
  line L53 (-422.6941, 18.1014) -> (-432.6941, 18.1014)
  line L54 (-432.6941, 18.1014) -> (-432.6941, -11.8986)
  line L55 (-432.6941, -11.8986) -> (-422.6941, -11.8986)
  arc A20 (-422.6941, -16.8986) -> (-422.6941, -11.8986) centre (-422.6941, -14.3986) ccw
  line L56 (-422.6941, -16.8986) -> (-422.6941, -114.3986)
  arc A21 (-422.6941, -119.3986) -> (-422.6941, -114.3986) centre (-422.6941, -116.8986) ccw
  line L57 (-422.6941, -119.3986) -> (-432.6941, -119.3986)
  line L58 (-432.6941, -119.3986) -> (-432.6941, -149.3986)
  line L59 (-432.6941, -149.3986) -> (-422.6941, -149.3986)
  arc A22 (-422.6941, -154.3986) -> (-422.6941, -149.3986) centre (-422.6941, -151.8986) ccw
  line L60 (-422.6941, -154.3986) -> (-422.6941, -246.8986)
  line L61 (-422.6941, -246.8986) -> (-392.6941, -246.8986)
  circle A23 centre (-200.3622, -246.9544) radius 2.5
  dimension "d314" = 5
  constraint coincident L7.end A23
  measures "d314" diameter of A23
extrude "Extrude34" cut sketch "Sketch54" against normal blind 10 contours L7 A23 picked at (-200.2999, -246.1234) bodies 1
sketch "Sketch55" plane through (0, 0, -256.8986) normal (0, 0, -1) x (1, 0, 0)
  arc A0 (-172.6941, 0) -> (-177.6941, 0) centre (-175.1941, 0) ccw
  line L0 (-172.6941, 0) -> (-172.6941, -10)
  line L1 (-172.6941, -10) -> (-142.6941, -10)
  line L2 (-142.6941, -10) -> (-142.6941, 25)
  arc A1 (-142.6941, 30) -> (-142.6941, 25) centre (-142.6941, 27.5) ccw
  line L3 (-142.6941, 30) -> (-132.6941, 30)
  line L4 (-132.6941, 30) -> (-132.6941, 60)
  line L5 (-132.6941, 60) -> (-142.6941, 60)
  arc A2 (-142.6941, 65) -> (-142.6941, 60) centre (-142.6941, 62.5) ccw
  line L6 (-142.6941, 65) -> (-142.6941, 100)
  line L7 (-142.6941, 100) -> (-422.6941, 100)
  line L8 (-422.6941, 100) -> (-422.6941, 65)
  arc A3 (-422.6941, 60) -> (-422.6941, 65) centre (-422.6941, 62.5) ccw
  line L9 (-422.6941, 60) -> (-432.6941, 60)
  line L10 (-432.6941, 60) -> (-432.6941, 30)
  line L11 (-432.6941, 30) -> (-422.6941, 30)
  arc A4 (-422.6941, 25) -> (-422.6941, 30) centre (-422.6941, 27.5) ccw
  line L12 (-422.6941, 25) -> (-422.6941, -10)
  line L13 (-422.6941, -10) -> (-392.6941, -10)
  line L14 (-392.6941, -10) -> (-392.6941, 0)
  arc A5 (-387.6941, 0) -> (-392.6941, 0) centre (-390.1941, 0) ccw
  line L15 (-387.6941, 0) -> (-367.694, 0)
  arc A6 (-362.6941, 0) -> (-367.694, 0) centre (-365.1941, 0.0132) ccw
  line L16 (-362.6941, 0) -> (-362.6941, -10)
  line L17 (-362.6941, -10) -> (-202.6941, -10)
  line L18 (-202.6941, -10) -> (-202.6941, 0)
  arc A7 (-197.6941, 0) -> (-202.6941, 0) centre (-200.1941, 0) ccw
  line L19 (-197.6941, 0) -> (-177.6941, 0)
  line L20 (-232.6941, 30) -> (-332.6941, 30)
  line L21 (-332.6941, 30) -> (-332.6941, 80)
  line L22 (-332.6941, 80) -> (-232.6941, 80)
  line L23 (-232.6941, 80) -> (-232.6941, 30)
  dimension "d317" = 100
  dimension "d318" = 50
  constraint horizontal L20
  constraint vertical L21
  constraint horizontal L22
  constraint vertical L23
  measures "d317" distance of L20.start L20.end
  measures "d318" distance of L20.start L22.end
extrude "Extrude35" cut sketch "Sketch55" against normal blind 10 contours L20 L21 L22 L23 bodies 8
sketch "Sketch56" plane through (0, -100, 0) normal (0, -1, 0) x (1, 0, 0)
  line L0 (-432.6941, 273.6512) -> (-432.6941, -256.3488)
  line L1 (-432.6941, -256.3488) -> (-422.6941, -256.3488)
  line L2 (-422.6941, -256.3488) -> (-422.6941, 273.6512)
  line L3 (-422.6941, 273.6512) -> (-432.6941, 273.6512)
  line L4 (-432.6941, 273.6512) -> (-132.6941, 273.6512)
  line L5 (-132.6941, 273.6512) -> (-132.6941, -256.3488)
  line L6 (-132.6941, -256.3488) -> (-432.6941, -256.3488)
  line L7 (-432.6941, -256.3488) -> (-432.6941, 273.6512)
  line L8 (-364.8822, 97.6075) -> (-199.8822, 97.6075)
  line L9 (-199.8822, 97.6075) -> (-199.8822, -67.3925)
  line L10 (-199.8822, -67.3925) -> (-364.8822, -67.3925)
  line L11 (-364.8822, -67.3925) -> (-364.8822, 97.6075)
  dimension "d321" = 300
  dimension "d322" = 530
  dimension "d323" = 165
  dimension "d324" = 165
  constraint horizontal L4
  constraint vertical L5
  constraint horizontal L6
  constraint vertical L7
  constraint coincident L0.start L3.end
  constraint horizontal L8
  constraint vertical L9
  constraint horizontal L10
  constraint vertical L11
  measures "d321" distance of L0.start L4.end
  measures "d322" distance of L0.start L0.end
  measures "d323" distance of L8.start L8.end
  measures "d324" distance of L8.start L10.end
extrude "Extrude36" add sketch "Sketch56" along normal blind 10 separate body contours L2 L4 L5 L6 makes body 9
sketch "Sketch57" plane through (0, 0, 0) normal (0, -1, 0) x (1, 0, 0)
sketch "Sketch58" plane through (0, -110, 0) normal (0, -1, 0) x (1, 0, 0)
  line L0 (-199.8822, -67.3925) -> (-364.8822, -67.3925)
  line L1 (-364.8822, -67.3925) -> (-364.8822, 97.6075)
  line L2 (-364.8822, 97.6075) -> (-199.8822, 97.6075)
  line L3 (-199.8822, 97.6075) -> (-199.8822, -67.3925)
  line L4 (-132.6941, -256.3488) -> (-132.6941, 273.6512)
  line L5 (-132.6941, 273.6512) -> (-422.6941, 273.6512)
  line L6 (-422.6941, 273.6512) -> (-422.6941, -256.3488)
  line L7 (-422.6941, -256.3488) -> (-132.6941, -256.3488)
  line L8 (-432.6941, 273.6512) -> (-422.6941, 273.6512)
  line L9 (-422.6941, 273.6512) -> (-422.6941, -266.3488)
  line L10 (-422.6941, -266.3488) -> (-432.6941, -266.3488)
  line L11 (-432.6941, -266.3488) -> (-432.6941, 273.6512)
  dimension "d327" = 10
  dimension "d328" = 540
  constraint horizontal L8
  constraint vertical L9
  constraint horizontal L10
  constraint vertical L11
  constraint coincident L5.end L6.start
  measures "d327" distance of L8.start L5.end
  measures "d328" distance of L8.start L10.end
extrude "Extrude37" add sketch "Sketch58" against normal blind 10 contours L6 L8 L9 L10 L11 bodies 9
sketch "Sketch59" plane through (0, -110, 0) normal (0, -1, 0) x (1, 0, 0)
  line L0 (-199.8822, -67.3925) -> (-364.8822, -67.3925)
  line L1 (-364.8822, -67.3925) -> (-364.8822, 97.6075)
  line L2 (-364.8822, 97.6075) -> (-199.8822, 97.6075)
  line L3 (-199.8822, 97.6075) -> (-199.8822, -67.3925)
  line L4 (-132.6941, -256.3488) -> (-132.6941, 273.6512)
  line L5 (-132.6941, 273.6512) -> (-432.6941, 273.6512)
  line L6 (-432.6941, 273.6512) -> (-432.6941, -266.3488)
  line L7 (-432.6941, -266.3488) -> (-422.6941, -266.3488)
  line L8 (-422.6941, -266.3488) -> (-422.6941, -256.3488)
  line L9 (-422.6941, -256.3488) -> (-132.6941, -256.3488)
  line L10 (-422.6941, -266.3488) -> (-432.6941, -266.3488)
  line L11 (-432.6941, -266.3488) -> (-432.6941, -256.3488)
  line L12 (-432.6941, -256.3488) -> (-422.6941, -256.3488)
  line L13 (-422.6941, -256.3488) -> (-422.6941, -266.3488)
  dimension "d331" = 10
  constraint horizontal L10
  constraint vertical L11
  constraint horizontal L12
  constraint vertical L13
  constraint coincident L6 L11.end
  constraint coincident L7.end L8.start
  measures "d331" distance of L7.end L8.end
extrude "Extrude38" cut sketch "Sketch59" against normal blind 10 contours L6 L7 L8 L10 L11 L12 L13 bodies 9